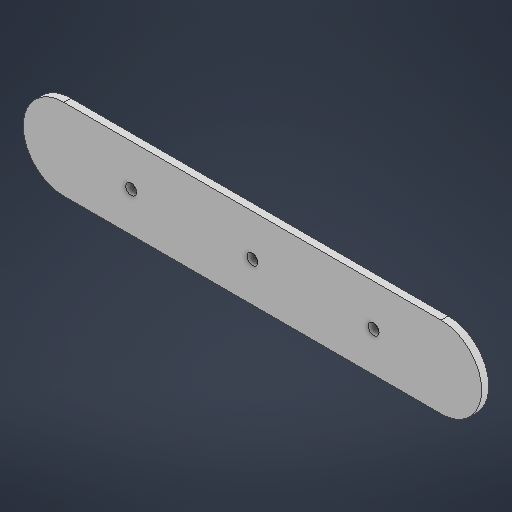
# Autodesk Inventor part: AMR_Handle_Flap
Saved by Autodesk Inventor 2026.2 (Build 302298010, 298A)
## iProperties
Created: 2026-03-27
Part Number: AMR_Handle_Flap
Material: Generic
Document SubType Name: Modeling
Designer: Srishanth Dhondy
Density: 1 g/cm^3
Appearance: Default
Author: Srishanth Dhondy
Autodesk Inventor part; units mm, degrees
ref_plane "YZ Plane" through (0, 0, 0) normal (1, 0, 0) x (0, 1, 0)
ref_plane "XZ Plane" through (0, 0, 0) normal (0, 1, 0) x (-1, 0, 0)
ref_plane "XY Plane" through (0, 0, 0) normal (0, 0, 1) x (1, 0, 0)
sketch "Sketch1" plane through (0, 0, 0) normal (0, 0, 1) x (1, 0, 0)
  line L0 (-79, 0) -> (79, 0) construction
  line L1 (-79, -17) -> (79, -17)
  line L2 (79, 17) -> (-79, 17)
  arc A0 (-79, 17) -> (-79, -17) centre (-79, 0) ccw
  arc A1 (79, -17) -> (79, 17) centre (79, 0) ccw
  point P0 (0, 0)
  dimension "d0" = 79
  dimension "d1" = 34
  constraints: 8 end point, 4 point on circle, 4 tangent, 2 centre point, 1 horizontal, 1 midpoint, 1 parallel
  measures "d0" distance of point (0, 0) L0.end
  measures "d1" diameter of A1
extrude "Extrusion1" add sketch "Sketch1" along normal blind 3
sketch "Sketch2" plane through (0, 0, 3) normal (0, 0, 1) x (1, 0, 0)
  line L0 (63.5, 11.5) -> (-63.5, 11.5)
  line L1 (-63.5, 11.5) -> (-63.5, -11.5)
  line L2 (-63.5, -11.5) -> (63.5, -11.5)
  line L3 (63.5, -11.5) -> (63.5, 11.5)
  line L4 (63.5, 11.5) -> (-63.5, -11.5) construction
  line L5 (-63.5, 11.5) -> (63.5, -11.5) construction
  line L6 (-63.5, 0) -> (63.5, 0)
  circle A0 centre (-50.8, -0.4) radius 2.25
  circle A1 centre (50.8, -0.4) radius 2.25
  circle A2 centre (0, -0.4) radius 2.25
  point P0 (0, 0)
  dimension "d4" = 23
  dimension "d5" = 4.5
  dimension "d6" = 4.5
  dimension "d7" = 4.5
  constraints: 14 end point, 8 coincident, 3 centre point, 2 midpoint, 2 parallel, 2 perpendicular, 1 horizontal
  measures "d4" distance of L1.end L0.end
  measures "d5" diameter of A0
  measures "d6" diameter of A1
  measures "d7" diameter of A2
extrude "Extrusion2" cut sketch "Sketch2" against normal through all contours A1 L6 | L6 A1 | A0 L6 | L6 A0 | A2 L6 | L6 A2
body "Solid1"
